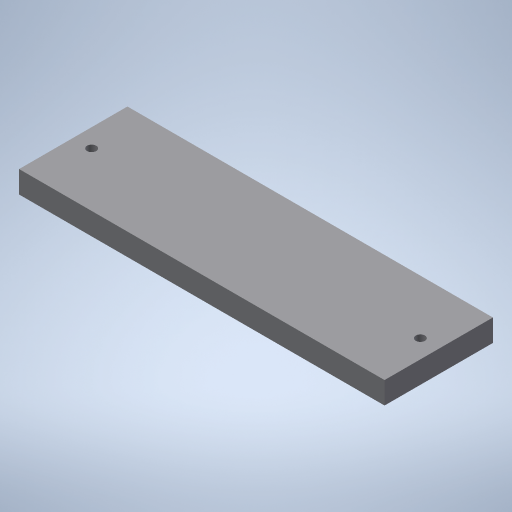
# Autodesk Inventor part: krab1
Saved by Autodesk Inventor 2023 (Build 270158000, 158)
## iProperties
Created: 2024-03-18
Part Number: krab1
Material: Všeobecné
Document SubType Name: Modeling
Designer: sok
Density: 1 g/cm^3
Appearance: Výchozí
Author: sok
Autodesk Inventor part; units mm, degrees
ref_plane "YZ Plane" through (0, 0, 0) normal (1, 0, 0) x (0, 1, 0)
ref_plane "XZ Plane" through (0, 0, 0) normal (0, 1, 0) x (-1, 0, 0)
ref_plane "Pracovní rovina11" through (0, 0, 164) normal (0, 0, 1) x (1, 0, 0)
sketch "Náčrt11" plane through (0, 0, 164) normal (0, 0, 1) x (1, 0, 0)
  line L0 (-0.5, -50.5) -> (190.5, -50.5)
  line L1 (190.5, -50.5) -> (190.5, 0.5)
  line L2 (190.5, 0.5) -> (-0.5, 0.5)
  line L3 (-0.5, 0.5) -> (-0.5, -50.5)
  line L4 (0, 0) -> (0, -50) projected
  line L5 (190, -50) -> (190, 0) projected
  line L6 (190, 0) -> (0, 0) projected
  line L7 (182, -50) -> (58, -50) projected
  line L8 (-4.5, 4.5) -> (194.5, 4.5)
  line L9 (194.5, 4.5) -> (194.5, -54.5)
  line L10 (194.5, -54.5) -> (-4.5, -54.5)
  line L11 (-4.5, -54.5) -> (-4.5, 4.5)
  dimension "d43" = 0.5
  dimension "d44" = 0.5
  dimension "d45" = 0.5
  dimension "d46" = 0.5
  dimension "d47" = 4
  constraints: 16 end point, 4 parallel, 2 perpendicular, 1 horizontal, 3 other
  measures "d43" distance between parallel lines of L4 L3
  measures "d44" distance between parallel lines of L1 L5
  measures "d45" distance between parallel lines of L6 L2
  measures "d46" distance between parallel lines of L0 L7
  measures "d47" distance between parallel lines of L2 L8
extrude "Vysunutí11" add sketch "Náčrt11" against normal blind 8
sketch "Náčrt12" plane through (0, 0, 164) normal (0, 0, 1) x (1, 0, 0)
  line L0 (-4.5, 4.5) -> (-4.5, -54.5) projected
  line L1 (194.5, 4.5) -> (-4.5, 4.5) projected
  line L2 (194.5, -54.5) -> (194.5, 4.5) projected
  line L3 (-4.5, -54.5) -> (194.5, -54.5) projected
  point P0 (0, 0)
extrude "Vysunutí12" add sketch "Náčrt12" along normal blind 4
sketch "Náčrt13" plane through (0, 0, 168) normal (0, 0, 1) x (1, 0, 0)
  circle A0 centre (5.5, -25) radius 2.5
  circle A1 centre (184.5, -25) radius 2.5
  line L0 (-4.5, -54.5) -> (194.5, -54.5) projected
  line L1 (194.5, 4.5) -> (-4.5, 4.5) projected
  line L2 (-4.5, 4.5) -> (-4.5, -54.5) projected
  line L3 (194.5, -54.5) -> (194.5, 4.5) projected
  point P0 (0, 0)
  dimension "d52" = 5
  dimension "d53" = 5
  dimension "d54" = 59
  dimension "d55" = 29.5
  dimension "d56" = 29.5
  dimension "d57" = 10
  dimension "d58" = 10
  constraints: 2 centre point
  measures "d52" diameter of A0
  measures "d53" diameter of A1
  measures "d54" distance between parallel lines of L0 L1
  measures "d55" distance from line of A0.centre L1
  measures "d56" distance from line of A1.centre L1
  measures "d57" distance from line of A0.centre L2
  measures "d58" distance from line of L3 A1.centre
extrude "Vysunutí13" cut sketch "Náčrt13" against normal through all contours A0 | A1
sketch "Náčrt14" plane through (-4.5, 4.5, 156) normal (0, 1, 0) x (1, 0, 0)
  line L0 (4, -8) -> (4, 0) projected
  line L1 (195, -8) -> (195, 0) projected
  line L2 (4, -8) -> (195, -8) projected
  line L3 (0, 0) -> (199, 0) projected
  point P0 (4.5, 156)
extrude "Vysunutí14" cut sketch "Náčrt14" against normal up to surface (4 mm away)
